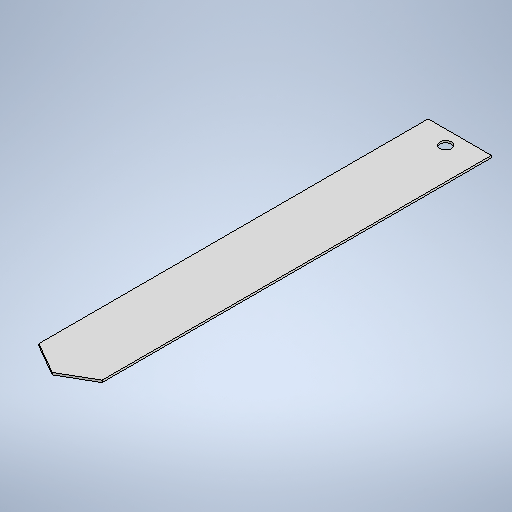
# Autodesk Inventor part: SLM 1696 leg floor pattern
Saved by Autodesk Inventor 2026.2 (Build 302298010, 298A)
## iProperties
Created: 2025-02-20
Part Number: SLM 1696 leg floor pattern
Material: Stainless Steel
Document SubType Name: Sheet Metal
Designer: user
Mass: 1021.57 g
Surface Area: 887.582 cm^2
Volume: 127.696 cm^3
Density: 8 g/cm^3
Sheet Metal Rule: AISI304 3mm Die 32
Sheet Metal Width: 90,000 mm
Sheet Metal Length: 580,000 mm
Sheet Metal Area: 52200,000 mm^2
Appearance: Default
Flat Pattern Width: 9 cm
Flat Pattern Length: 58 cm
Flat Pattern Area: 522 cm^2
Author: user
Autodesk Inventor part; units mm, degrees
ref_plane "YZ Plane" through (0, 0, 0) normal (1, 0, 0) x (0, 1, 0)
ref_plane "XZ Plane" through (0, 0, 0) normal (0, 1, 0) x (-1, 0, 0)
ref_plane "XY Plane" through (0, 0, 0) normal (0, 0, 1) x (1, 0, 0)
sketch "Sketch6" plane through (0, 0, 0) normal (0, 0, 1) x (1, 0, 0)
  line L0 (0, 0) -> (45, 25.9808)
  line L1 (0, 0) -> (-45, 25.9808)
  line L2 (0, 0) -> (0, 560)
  line L3 (-45, 25.9808) -> (45, 25.9808)
  line L4 (45, 25.9808) -> (45, 580)
  line L5 (45, 580) -> (-45, 580)
  line L6 (-45, 580) -> (-45, 25.9808)
  circle A0 centre (0, 560) radius 8.5
  circle A1 centre (0, 0) radius 560 construction
  circle A2 centre (0, 0) radius 580 construction
  dimension "d44" = 1120
  dimension "d40" = 120
  dimension "d42" = 90
  dimension "d43" = 17
  dimension "d45" = 1160
  dimension "d47" = 20
  measures "d40" angle of L0 L1
  measures "d42" distance between parallel lines of L4 L6
  measures "d43" diameter of A0
  measures "d45" diameter of A2
extrude "Plate3" add sketch "Sketch6" along normal blind 3
equation "\"d46\" = Thickness"
equation "\"BendReliefWidth\" = Thickness"
equation "\"BendReliefDepth\" = 0.5 * Thickness"
equation "\"CornerReliefSize\" = 4 * Thickness"
equation "\"MinimumRemnant\" = 2 * Thickness"
equation "\"TransitionRadius\" = BendRadius"
equation "\"JacobiRadiusSize\" = BendRadius"
equation "\"GapSize\" = Thickness"
equation "\"Thickness\" = 3"
equation "\"BendRadius\" = 5"
body "Solid2"
